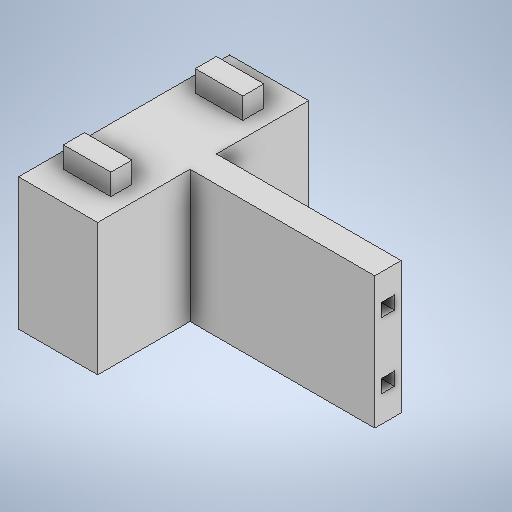
# Autodesk Inventor part: Hurdle Split
Saved by Autodesk Inventor 2026.1 (Build 301233000, 233)
## iProperties
Created: 2026-01-06
Part Number: Hurdle Split
Material: Generic
Document SubType Name: Modeling
Designer: User
Density: 1 g/cm^3
Appearance: Default
Author: User
Autodesk Inventor part; units mm, degrees
ref_plane "YZ Plane" through (0, 0, 0) normal (1, 0, 0) x (0, 1, 0)
ref_plane "XZ Plane" through (0, 0, 0) normal (0, 1, 0) x (-1, 0, 0)
ref_plane "XY Plane" through (0, 0, 0) normal (0, 0, 1) x (1, 0, 0)
sketch "Sketch1" plane through (0, 0, 0) normal (0, 1, 0) x (-1, 0, 0)
  line L0 (-10, -55) -> (-160, -55)
  line L1 (-160, -55) -> (-160, -45)
  line L2 (-160, -45) -> (-10, -45)
  line L3 (-10, -45) -> (-10, -55)
  line L4 (10, -55) -> (80, -55)
  line L5 (80, -55) -> (80, -90)
  line L6 (80, -90) -> (110, -90)
  line L7 (110, -90) -> (110, -10)
  line L8 (110, -10) -> (80, -10)
  line L9 (80, -10) -> (80, -45)
  line L10 (80, -45) -> (10, -45)
  line L11 (10, -45) -> (10, -55)
  line L12 (0, -122.2654) -> (0, -189.4683)
  line L13 (-10, 55) -> (-10, 45)
  line L14 (10, 55) -> (10, 45)
  line L15 (80, 10) -> (110, 10)
  line L16 (10, 45) -> (80, 45)
  line L17 (80, 45) -> (80, 10)
  line L18 (80, 55) -> (10, 55)
  line L19 (80, 90) -> (80, 55)
  line L20 (110, 10) -> (110, 90)
  line L21 (110, 90) -> (80, 90)
  line L22 (-160, 55) -> (-10, 55)
  line L23 (-160, 45) -> (-160, 55)
  line L24 (-10, 45) -> (-160, 45)
  point P0 (0, 0)
  dimension "d0" = 10
  dimension "d1" = 80
  dimension "d2" = 10
  dimension "d4" = 30
  dimension "d5" = 30
  dimension "d6" = 35
  dimension "d7" = 35
  dimension "d8" = 45
  dimension "d9" = 10
  dimension "d10" = 10
  dimension "d11" = 150
  dimension "d12" = 100
  dimension "d13" = 0
  dimension "d16" = 100
  constraints: 50 end point, 6 perpendicular, 4 parallel, 2 horizontal, 2 vertical, 24 other
  measures "d0" distance from line of point (0, 0) L8
  measures "d1" distance of L6.end L7.end
  measures "d2" distance from line of point (0, 0) L11
  measures "d4" distance of L5.end L6.end
  measures "d5" distance of L7.end L8.end
  measures "d6" distance of L8.end L9.end
  measures "d7" distance of L4.end L5.end
  measures "d8" distance from line of point (0, 0) L2
  measures "d9" distance of L2.end L0.start
  measures "d10" distance from line of point (0, 0) L3
  measures "d11" distance of L0.start L0.end
  measures "d12" distance between parallel lines of L11 L7
  measures "d13" distance from line of point (0, 0) L12
  measures "d16" distance of L0.start L13.end
extrude "Extrusion1" add sketch "Sketch1" along normal blind 50
sketch "Sketch2" plane through (160, 0, 55) normal (1, 0, 0) x (0, 0, -1)
  line L0 (2.5, 40) -> (7.5, 40)
  line L1 (7.5, 40) -> (7.5, 35)
  line L2 (7.5, 35) -> (2.5, 35)
  line L3 (2.5, 35) -> (2.5, 40)
  line L4 (0, 50) -> (10, 50) projected
  line L5 (10, 0) -> (10, 50) projected
  line L6 (2.5, 15) -> (7.5, 15)
  line L7 (7.5, 15) -> (7.5, 10)
  line L8 (7.5, 10) -> (2.5, 10)
  line L9 (2.5, 10) -> (2.5, 15)
  line L10 (102.5, 40) -> (107.5, 40)
  line L11 (107.5, 40) -> (107.5, 35)
  line L12 (107.5, 35) -> (102.5, 35)
  line L13 (102.5, 35) -> (102.5, 40)
  line L14 (102.5, 15) -> (107.5, 15)
  line L15 (107.5, 15) -> (107.5, 10)
  line L16 (107.5, 10) -> (102.5, 10)
  line L17 (102.5, 10) -> (102.5, 15)
  point P0 (55, 0)
  dimension "d23" = 10
  dimension "d24" = 5
  dimension "d25" = 2.5
  dimension "d26" = 5
  dimension "d29" = 25
  dimension "d32" = 100
  constraints: 32 end point, 2 horizontal, 2 parallel, 1 perpendicular, 1 vertical, 24 other
  measures "d23" distance between parallel lines of L4 L0
  measures "d24" distance of L2.end L0.start
  measures "d25" distance between parallel lines of L5 L1
  measures "d26" distance of L1.end L2.end
  measures "d29" distance of L0.start L6.start
  measures "d32" distance of L0.start L10.start
extrude "Extrusion2" cut sketch "Sketch2" against normal blind 200
sketch "Sketch3" plane through (0, 50, 0) normal (0, 1, 0) x (1, 0, 0)
  line L0 (-105, -20) -> (-85, -20)
  line L1 (-85, -20) -> (-85, -30)
  line L2 (-85, -30) -> (-105, -30)
  line L3 (-105, -30) -> (-105, -20)
  line L4 (-110, -10) -> (-110, -90) projected
  line L5 (-105, -70) -> (-85, -70)
  line L6 (-85, -70) -> (-85, -80)
  line L7 (-85, -80) -> (-105, -80)
  line L8 (-105, -80) -> (-105, -70)
  line L9 (-105, 80) -> (-85, 80)
  line L10 (-85, 80) -> (-85, 70)
  line L11 (-85, 70) -> (-105, 70)
  line L12 (-105, 70) -> (-105, 80)
  line L13 (-105, 30) -> (-85, 30)
  line L14 (-85, 30) -> (-85, 20)
  line L15 (-85, 20) -> (-105, 20)
  line L16 (-105, 20) -> (-105, 30)
  point P0 (0, 0)
  dimension "d37" = 20
  dimension "d38" = 10
  dimension "d39" = 20
  dimension "d40" = 85
  dimension "d43" = 50
  dimension "d46" = 100
  constraints: 32 end point, 2 parallel, 2 vertical, 1 horizontal, 1 perpendicular, 24 other
  measures "d37" distance from line of L0 point (0, 0)
  measures "d38" distance of L2.end L0.start
  measures "d39" distance of L0.start L0.end
  measures "d40" distance from line of point (0, 0) L1
  measures "d43" distance of L0.start L5.start
  measures "d46" distance of L0.start L9.start
extrude "Extrusion3" add sketch "Sketch3" along normal blind 8
sketch "Sketch4" plane through (0, 0, 0) normal (0, -1, 0) x (1, 0, 0)
  line L0 (-105, -70) -> (-85, -70) projected
  line L1 (-85, -70) -> (-85, -80) projected
  line L2 (-85, -80) -> (-105, -80) projected
  line L3 (-105, -80) -> (-105, -70) projected
  line L4 (-105, -20) -> (-85, -20) projected
  line L5 (-85, -20) -> (-85, -30) projected
  line L6 (-85, -30) -> (-105, -30) projected
  line L7 (-105, -30) -> (-105, -20) projected
  line L8 (-105, 30) -> (-85, 30) projected
  line L9 (-85, 30) -> (-85, 20) projected
  line L10 (-85, 20) -> (-105, 20) projected
  line L11 (-105, 20) -> (-105, 30) projected
  line L12 (-105, 80) -> (-85, 80) projected
  line L13 (-85, 80) -> (-85, 70) projected
  line L14 (-85, 70) -> (-105, 70) projected
  line L15 (-105, 70) -> (-105, 80) projected
  line L16 (-85, 80) -> (-105, 80)
  line L17 (-105, 80) -> (-105, 70)
  line L18 (-105, 70) -> (-85, 70)
  line L19 (-85, 70) -> (-85, 80)
  line L20 (-85, 30) -> (-105, 30)
  line L21 (-105, 30) -> (-105, 20)
  line L22 (-105, 20) -> (-85, 20)
  line L23 (-85, 20) -> (-85, 30)
  line L24 (-85, -20) -> (-105, -20)
  line L25 (-105, -20) -> (-105, -30)
  line L26 (-105, -30) -> (-85, -30)
  line L27 (-85, -30) -> (-85, -20)
  line L28 (-85, -70) -> (-105, -70)
  line L29 (-105, -70) -> (-105, -80)
  line L30 (-105, -80) -> (-85, -80)
  line L31 (-85, -80) -> (-85, -70)
  point P0 (0, 0)
  constraints: 32 end point, 8 parallel, 4 horizontal, 4 perpendicular
extrude "Extrusion4" cut sketch "Sketch4" against normal blind 10
sketch "Sketch5" plane through (10, 0, 55) normal (0, 0, 1) x (1, 0, 0)
  line L0 (0, 0) -> (0, 50) projected
  line L1 (0, 50) -> (150, 50) projected
  line L2 (150, 0) -> (150, 50) projected
  line L3 (0, 0) -> (150, 0) projected
  line L4 (0, 35) -> (0, 40) projected
  line L5 (150, 35) -> (0, 35) projected
  line L6 (150, 40) -> (150, 35) projected
  line L7 (150, 40) -> (0, 40) projected
  line L8 (0, 10) -> (0, 15) projected
  line L9 (150, 10) -> (0, 10) projected
  line L10 (150, 15) -> (150, 10) projected
  line L11 (150, 15) -> (0, 15) projected
  line L12 (10, 40) -> (140, 40)
  line L13 (140, 40) -> (140, 35)
  line L14 (140, 35) -> (10, 35)
  line L15 (10, 35) -> (10, 40)
  line L16 (10, 15) -> (140, 15)
  line L17 (140, 15) -> (140, 10)
  line L18 (140, 10) -> (10, 10)
  line L19 (10, 10) -> (10, 15)
  point P0 (-10, 0)
  point P1 (10, 10)
  dimension "d53" = 10
  dimension "d54" = 10
  dimension "d55" = 10
  dimension "d56" = 10
  constraints: 16 end point, 4 parallel, 4 point on line, 2 horizontal, 2 perpendicular
  measures "d53" distance between parallel lines of L0 L15
  measures "d54" distance between parallel lines of L6 L13
  measures "d55" distance between parallel lines of L2 L17
  measures "d56" distance between parallel lines of L8 L19
extrude "Extrusion5" add sketch "Sketch5" against normal blind 10 contours L19 L11 L17 L9 | L15 L7 L13 L5
sketch "Sketch6" plane through (160, 0, -55) normal (0, 0, -1) x (-1, 0, 0)
  line L0 (150, 40) -> (150, 35) projected
  line L1 (0, 40) -> (150, 40) projected
  line L2 (0, 35) -> (0, 40) projected
  line L3 (0, 35) -> (150, 35) projected
  line L4 (150, 15) -> (150, 10) projected
  line L5 (0, 15) -> (150, 15) projected
  line L6 (0, 10) -> (0, 15) projected
  line L7 (0, 10) -> (150, 10) projected
  line L8 (10, 40) -> (140, 40)
  line L9 (140, 40) -> (140, 35)
  line L10 (140, 35) -> (10, 35)
  line L11 (10, 35) -> (10, 40)
  line L12 (10, 15) -> (140, 15)
  line L13 (140, 15) -> (140, 10)
  line L14 (140, 10) -> (10, 10)
  line L15 (10, 10) -> (10, 15)
  point P0 (160, 0)
  point P1 (140, 37.5)
  point P2 (10, 10)
  dimension "d59" = 10
  dimension "d60" = 10
  dimension "d61" = 10
  dimension "d62" = 10
  constraints: 16 end point, 4 parallel, 4 point on line, 2 horizontal, 2 perpendicular, 1 midpoint
  measures "d59" distance between parallel lines of L2 L11
  measures "d60" distance between parallel lines of L6 L15
  measures "d61" distance between parallel lines of L4 L13
  measures "d62" distance from line of L0 point (140, 37.5)
extrude "Extrusion6" add sketch "Sketch6" against normal blind 10 contours L9 L3 L11 L1 | L13 L7 L15 L5
sketch "Sketch7" plane through (0, 58, 0) normal (0, 1, 0) x (1, 0, 0)
  line L0 (-105, -80) -> (-85, -80) projected
  line L1 (-85, -80) -> (-85, -70) projected
  line L2 (-85, -70) -> (-105, -70) projected
  line L3 (-105, -70) -> (-105, -80) projected
  line L4 (-105, -30) -> (-85, -30) projected
  line L5 (-85, -30) -> (-85, -20) projected
  line L6 (-85, -20) -> (-105, -20) projected
  line L7 (-105, -20) -> (-105, -30) projected
  line L8 (-105, 20) -> (-85, 20) projected
  line L9 (-85, 20) -> (-85, 30) projected
  line L10 (-85, 30) -> (-105, 30) projected
  line L11 (-105, 30) -> (-105, 20) projected
  line L12 (-105, 70) -> (-85, 70) projected
  line L13 (-85, 70) -> (-85, 80) projected
  line L14 (-85, 80) -> (-105, 80) projected
  line L15 (-105, 80) -> (-105, 70) projected
  line L16 (-104, -79) -> (-86, -79)
  line L17 (-86, -79) -> (-86, -71)
  line L18 (-86, -71) -> (-104, -71)
  line L19 (-104, -71) -> (-104, -79)
  line L20 (-86, -21) -> (-104, -21)
  line L21 (-104, -21) -> (-104, -29)
  line L22 (-104, -29) -> (-86, -29)
  line L23 (-86, -29) -> (-86, -21)
  line L24 (-86, 29) -> (-104, 29)
  line L25 (-104, 29) -> (-104, 21)
  line L26 (-104, 21) -> (-86, 21)
  line L27 (-86, 21) -> (-86, 29)
  line L28 (-86, 79) -> (-104, 79)
  line L29 (-104, 79) -> (-104, 71)
  line L30 (-104, 71) -> (-86, 71)
  line L31 (-86, 71) -> (-86, 79)
  line L32 (-105, -80) -> (-85, -80)
  line L33 (-85, -80) -> (-85, -70)
  line L34 (-85, -70) -> (-105, -70)
  line L35 (-105, -70) -> (-105, -80)
  line L36 (-105, -30) -> (-85, -30)
  line L37 (-85, -30) -> (-85, -20)
  line L38 (-85, -20) -> (-105, -20)
  line L39 (-105, -20) -> (-105, -30)
  line L40 (-105, 20) -> (-85, 20)
  line L41 (-85, 20) -> (-85, 30)
  line L42 (-85, 30) -> (-105, 30)
  line L43 (-105, 30) -> (-105, 20)
  line L44 (-105, 70) -> (-85, 70)
  line L45 (-85, 70) -> (-85, 80)
  line L46 (-85, 80) -> (-105, 80)
  line L47 (-105, 80) -> (-105, 70)
  point P0 (0, 0)
  dimension "d65" = 1
  dimension "d66" = 1
  dimension "d67" = 1
  dimension "d68" = 1
  dimension "d71" = 50
  dimension "d74" = 100
  constraints: 64 end point, 10 parallel, 5 horizontal, 5 perpendicular, 2 vertical, 24 other
  measures "d65" distance between parallel lines of L0 L16
  measures "d66" distance between parallel lines of L2 L18
  measures "d67" distance between parallel lines of L3 L19
  measures "d68" distance between parallel lines of L1 L17
  measures "d71" distance of L17.end L20.start
  measures "d74" distance of L17.end L24.start
extrude "Extrusion7" cut sketch "Sketch7" against normal blind 8
sketch "Sketch8" plane through (-80, 0, 55) normal (0, 0, 1) x (1, 0, 0)
  line L0 (70, 40) -> (70, 35) projected
  line L1 (70, 40) -> (40, 40) projected
  line L2 (40, 40) -> (40, 35) projected
  line L3 (70, 35) -> (40, 35) projected
  line L4 (70, 15) -> (70, 10) projected
  line L5 (70, 15) -> (40, 15) projected
  line L6 (40, 15) -> (40, 10) projected
  line L7 (70, 10) -> (40, 10) projected
  line L8 (40, 40) -> (60, 40)
  line L9 (60, 40) -> (60, 35)
  line L10 (60, 35) -> (40, 35)
  line L11 (40, 35) -> (40, 40)
  line L12 (40, 15) -> (60, 15)
  line L13 (60, 15) -> (60, 10)
  line L14 (60, 10) -> (40, 10)
  line L15 (40, 10) -> (40, 15)
  point P0 (80, 0)
  point P1 (60, 15)
  point P2 (60, 40)
  dimension "d79" = 10
  dimension "d80" = 10
  constraints: 16 end point, 4 parallel, 2 horizontal, 2 perpendicular, 2 point on line
  measures "d79" distance from line of L0 L9.end
  measures "d80" distance between parallel lines of L4 L13
extrude "Extrusion8" add sketch "Sketch8" against normal blind 10 contours L9 L3 L2 L1 | L13 L7 L6 L5
sketch "Sketch9" plane through (-10, 0, -55) normal (0, 0, -1) x (-1, 0, 0)
  line L0 (0, 35) -> (0, 40) projected
  line L1 (0, 35) -> (30, 35) projected
  line L2 (30, 35) -> (30, 40) projected
  line L3 (0, 40) -> (30, 40) projected
  line L4 (0, 10) -> (0, 15) projected
  line L5 (0, 10) -> (30, 10) projected
  line L6 (30, 10) -> (30, 15) projected
  line L7 (0, 15) -> (30, 15) projected
  line L8 (30, 40) -> (10, 40)
  line L9 (10, 40) -> (10, 10)
  line L10 (10, 10) -> (30, 10)
  line L11 (30, 10) -> (30, 40)
  point P0 (-10, 0)
  point P1 (0, 37.5)
  dimension "d83" = 10
  constraints: 8 end point, 2 parallel, 1 horizontal, 1 midpoint, 1 perpendicular, 1 point on line
  measures "d83" distance from line of point (0, 37.5) L9
extrude "Extrusion9" add sketch "Sketch9" against normal blind 10 contours L9 L3 L2 L1 | L1 L11 L7 L9 | L7 L6 L5 L9
sketch "Sketch10" plane through (0, 58, 0) normal (0, 1, 0) x (1, 0, 0)
  line L0 (-140, 100) -> (-140, 0)
  line L1 (-140, 0) -> (0, 0)
  line L2 (0, 0) -> (0, -100)
  line L3 (0, -100) -> (180, -100)
  line L4 (180, -100) -> (180, 100)
  line L5 (180, 100) -> (-140, 100)
  dimension "d86" = 100
  dimension "d87" = 320
  dimension "d88" = 200
  dimension "d89" = 180
  constraints: 12 end point, 5 perpendicular, 1 vertical
  measures "d86" distance of L0.start L0.end
  measures "d87" distance of L4.end L0.start
  measures "d88" distance of L3.end L4.end
  measures "d89" distance of L2.end L3.end
extrude "Extrusion10" cut sketch "Sketch10" against normal through all
body "Solid1"
